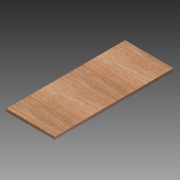
# Autodesk Inventor part: Left Mounting Board
Saved by Autodesk Inventor 2014 (Build 180170000, 170)
## iProperties
Created: 2016-02-04
Part Number: Left Mounting Board
Material: Generic
Document SubType Name: Modeling
Designer: zoldberg
Density: 1 g/cm^3
Appearance: Birch - Natural Polished
Author: zoldberg
Autodesk Inventor part; units mm, degrees
ref_plane "YZ Plane" through (0, 0, 0) normal (1, 0, 0) x (0, 1, 0)
ref_plane "XZ Plane" through (0, 0, 0) normal (0, 1, 0) x (-1, 0, 0)
ref_plane "XY Plane" through (0, 0, 0) normal (0, 0, 1) x (1, 0, 0)
sketch "Sketch1" plane through (0, 0, 0) normal (0, 0, 1) x (1, 0, 0)
  line L0 (-114.3, -25.4) -> (114.3, -25.4)
  line L1 (114.3, -25.4) -> (114.3, 25.4)
  line L2 (114.3, 25.4) -> (-114.3, 25.4)
  line L3 (-114.3, 25.4) -> (-114.3, -25.4)
  line L4 (-114.3, -25.4) -> (114.3, 25.4) construction
  line L5 (114.3, -25.4) -> (-114.3, 25.4) construction
  point P0 (0, 0)
  dimension "d0" = 228.6
  dimension "d1" = 50.8
  constraints: 12 end point, 2 midpoint, 2 parallel, 1 horizontal, 1 perpendicular
  measures "d0" distance of L2.end L1.end
  measures "d1" distance of L1.end L0.end
extrude "Extrusion1" add sketch "Sketch1" along normal blind 558.8
sketch "Sketch2" plane through (-114.3, 25.4, 0) normal (0, 1, 0) x (1, 0, 0)
  line L0 (228.6, 0) -> (0, 0) projected
  line L1 (0, 0) -> (0, -558.8) projected
  line L2 (228.6, -558.8) -> (0, -558.8) projected
  line L3 (228.6, 0) -> (228.6, -558.8) projected
  point P0 (114.3, 0)
extrude "Extrusion2" cut sketch "Sketch2" against normal blind 38.1
body "Solid1"
